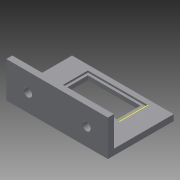
# Autodesk Inventor part: sampleholderdraft5
Saved by Autodesk Inventor 2014 SP1 (Build 180222100, 222)
## iProperties
Created: 2014-06-06
Part Number: sampleholderdraft5
Material: Generic
Document SubType Name: Modeling
Designer: miles90
Density: 1 g/cm^3
Appearance: Default
Author: miles90
Autodesk Inventor part; units mm, degrees
ref_plane "YZ Plane" through (0, 0, 0) normal (1, 0, 0) x (0, 1, 0)
ref_plane "XZ Plane" through (0, 0, 0) normal (0, 1, 0) x (-1, 0, 0)
ref_plane "XY Plane" through (0, 0, 0) normal (0, 0, 1) x (1, 0, 0)
sketch "Sketch1" plane through (0, 0, 0) normal (0, 1, 0) x (-1, 0, 0)
  line L0 (52.3087, -21.6726) -> (-32.6913, -21.6726)
  line L1 (-32.6913, -21.6726) -> (-32.6913, 38.3274)
  line L2 (-32.6913, 38.3274) -> (52.3087, 38.3274)
  line L3 (52.3087, 38.3274) -> (52.3087, -21.6726)
  dimension "d4" = 60
  dimension "d5" = 85
  constraints: 8 end point, 2 parallel, 1 horizontal, 1 perpendicular
  measures "d4" distance of L2.end L0.start
  measures "d5" distance of L0.start L0.end
extrude "Extrusion1" add sketch "Sketch1" along normal blind 20
sketch "Sketch2" plane through (0, 20, 0) normal (0, 1, 0) x (1, 0, 0)
  line L0 (32.6913, 21.6726) -> (-52.3087, 21.6726) projected
  line L1 (-52.3087, 21.6726) -> (-52.3087, -38.3274) projected
  line L2 (-52.3087, -38.3274) -> (32.6913, -38.3274) projected
  line L3 (32.6913, -38.3274) -> (32.6913, 21.6726) projected
  line L4 (-52.3087, 16.6726) -> (32.6913, 16.6726)
  line L5 (32.6913, 16.6726) -> (32.6913, -33.3274)
  line L6 (32.6913, -33.3274) -> (-52.3087, -33.3274)
  line L7 (-52.3087, -33.3274) -> (-52.3087, 16.6726)
  point P0 (0, 0)
  dimension "d8" = 0
  dimension "d9" = 0
  dimension "d10" = 5
  dimension "d11" = 5
  constraints: 8 end point, 2 parallel, 1 horizontal, 1 perpendicular
  measures "d8" distance between parallel lines of L1 L7
  measures "d9" distance between parallel lines of L5 L3
  measures "d10" distance between parallel lines of L6 L2
  measures "d11" distance between parallel lines of L0 L4
extrude "Extrusion2" cut sketch "Sketch2" against normal blind 15 contours L3 L6 L1 L4
sketch "Sketch3" plane through (0, 5, 0) normal (0, 1, 0) x (1, 0, 0)
  line L0 (-52.3087, 16.6726) -> (32.6913, 16.6726) projected
  line L1 (-52.3087, -33.3274) -> (-52.3087, 16.6726) projected
  line L2 (32.6913, -33.3274) -> (-52.3087, -33.3274) projected
  line L3 (32.6913, 16.6726) -> (32.6913, -33.3274) projected
  line L4 (-34.8087, 12.4226) -> (15.1913, 12.4226)
  line L5 (15.1913, 12.4226) -> (15.1913, -11.3274)
  line L6 (15.1913, -11.3274) -> (-34.8087, -11.3274)
  line L7 (-34.8087, -11.3274) -> (-34.8087, 12.4226)
  point P0 (0, 0)
  dimension "d14" = 17.5
  dimension "d15" = 17.5
  dimension "d16" = 4.25
  dimension "d17" = 22
  constraints: 8 end point, 2 parallel, 1 horizontal, 1 perpendicular
  measures "d14" distance between parallel lines of L3 L5
  measures "d15" distance between parallel lines of L1 L7
  measures "d16" distance between parallel lines of L4 L0
  measures "d17" distance between parallel lines of L6 L2
extrude "Extrusion3" cut sketch "Sketch3" against normal blind 1.5 contours L4 L5 L6 L7
sketch "Sketch4" plane through (0, 3.5, 0) normal (0, 1, 0) x (1, 0, 0)
  line L0 (-34.8087, 12.4226) -> (15.1913, 12.4226) projected
  line L1 (-34.8087, -11.3274) -> (-34.8087, 12.4226) projected
  line L2 (15.1913, -11.3274) -> (-34.8087, -11.3274) projected
  line L3 (15.1913, 12.4226) -> (15.1913, -11.3274) projected
  line L4 (-32.8087, 10.4226) -> (11.1913, 10.4226)
  line L5 (11.1913, 10.4226) -> (11.1913, -9.3274)
  line L6 (11.1913, -9.3274) -> (-32.8087, -9.3274)
  line L7 (-32.8087, -9.3274) -> (-32.8087, 10.4226)
  point P0 (0, 0)
  dimension "d20" = 2
  dimension "d21" = 2
  dimension "d22" = 2
  dimension "d23" = 4
  constraints: 8 end point, 2 parallel, 1 horizontal, 1 perpendicular
  measures "d20" distance between parallel lines of L1 L7
  measures "d21" distance between parallel lines of L0 L4
  measures "d22" distance between parallel lines of L2 L6
  measures "d23" distance between parallel lines of L3 L5
extrude "Extrusion4" cut sketch "Sketch4" against normal blind 1 contours L4 L5 L6 L7
sketch "Sketch5" plane through (0, 20, 0) normal (0, 1, 0) x (1, 0, 0)
  line L0 (32.6913, -33.3274) -> (-52.3087, -33.3274) projected
  line L1 (-52.3087, -33.3274) -> (-52.3087, -38.3274) projected
  line L2 (-52.3087, -38.3274) -> (32.6913, -38.3274) projected
  line L3 (32.6913, -38.3274) -> (32.6913, -33.3274) projected
  line L4 (-52.3087, -33.3274) -> (32.6913, -33.3274)
  line L5 (32.6913, -33.3274) -> (32.6913, -38.3274)
  line L6 (32.6913, -38.3274) -> (-52.3087, -38.3274)
  line L7 (-52.3087, -38.3274) -> (-52.3087, -33.3274)
  point P0 (0, 0)
  dimension "d26" = 0
  dimension "d27" = 0
  dimension "d28" = 0
  dimension "d29" = 0
  constraints: 8 end point, 2 parallel, 1 horizontal, 1 perpendicular
  measures "d26" distance between parallel lines of L0 L4
  measures "d27" distance between parallel lines of L2 L6
  measures "d28" distance between parallel lines of L3 L5
  measures "d29" distance between parallel lines of L1 L7
extrude "Extrusion5" add sketch "Sketch5" against normal blind 35
sketch "Sketch6" plane through (0, 20, 0) normal (0, 1, 0) x (1, 0, 0)
  line L0 (-52.3087, 16.6726) -> (32.6913, 16.6726) projected
  line L1 (32.6913, 16.6726) -> (32.6913, 21.6726) projected
  line L2 (32.6913, 21.6726) -> (-52.3087, 21.6726) projected
  line L3 (-52.3087, 21.6726) -> (-52.3087, 16.6726) projected
  line L4 (-52.3087, 21.6726) -> (32.6913, 21.6726)
  line L5 (32.6913, 21.6726) -> (32.6913, 16.6726)
  line L6 (32.6913, 16.6726) -> (-52.3087, 16.6726)
  line L7 (-52.3087, 16.6726) -> (-52.3087, 21.6726)
  point P0 (0, 0)
  dimension "d32" = 0
  dimension "d33" = 0
  dimension "d34" = 0
  dimension "d35" = 0
  constraints: 8 end point, 2 parallel, 1 horizontal, 1 perpendicular
  measures "d32" distance between parallel lines of L2 L4
  measures "d33" distance between parallel lines of L0 L6
  measures "d34" distance between parallel lines of L3 L7
  measures "d35" distance between parallel lines of L1 L5
extrude "Extrusion6" cut sketch "Sketch6" against normal blind 20
sketch "Sketch8" plane through (0, 20, 0) normal (0, 1, 0) x (1, 0, 0)
  line L0 (32.6913, -33.3274) -> (-52.3087, -33.3274) projected
  line L1 (-52.3087, -33.3274) -> (-52.3087, -38.3274) projected
  line L2 (-52.3087, -38.3274) -> (32.6913, -38.3274) projected
  line L3 (32.6913, -38.3274) -> (32.6913, -33.3274) projected
  line L4 (-52.3087, -33.3274) -> (32.6913, -33.3274)
  line L5 (32.6913, -33.3274) -> (32.6913, -38.3274)
  line L6 (32.6913, -38.3274) -> (-52.3087, -38.3274)
  line L7 (-52.3087, -38.3274) -> (-52.3087, -33.3274)
  point P0 (0, 0)
  dimension "d41" = 0
  dimension "d42" = 0
  dimension "d43" = 0
  dimension "d44" = 0
  constraints: 8 end point, 2 parallel, 1 horizontal, 1 perpendicular
  measures "d41" distance between parallel lines of L3 L5
  measures "d42" distance between parallel lines of L1 L7
  measures "d43" distance between parallel lines of L2 L6
  measures "d44" distance between parallel lines of L0 L4
extrude "Extrusion7" add sketch "Sketch8" along normal blind 10
sketch "Sketch9" plane through (0, -15, 0) normal (0, -1, 0) x (1, 0, 0)
  line L0 (-52.3087, 33.3274) -> (32.6913, 33.3274) projected
  line L1 (32.6913, 33.3274) -> (32.6913, 38.3274) projected
  line L2 (32.6913, 38.3274) -> (-52.3087, 38.3274) projected
  line L3 (-52.3087, 38.3274) -> (-52.3087, 33.3274) projected
  line L4 (-52.3087, 38.3274) -> (32.6913, 38.3274)
  line L5 (32.6913, 38.3274) -> (32.6913, 33.3274)
  line L6 (32.6913, 33.3274) -> (-52.3087, 33.3274)
  line L7 (-52.3087, 33.3274) -> (-52.3087, 38.3274)
  point P0 (0, 0)
  dimension "d47" = 0
  dimension "d48" = 0
  dimension "d49" = 0
  dimension "d50" = 0
  constraints: 8 end point, 2 parallel, 1 horizontal, 1 perpendicular
  measures "d47" distance between parallel lines of L2 L4
  measures "d48" distance between parallel lines of L3 L7
  measures "d49" distance between parallel lines of L0 L6
  measures "d50" distance between parallel lines of L1 L5
extrude "Extrusion8" add sketch "Sketch9" along normal blind 10
sketch "Sketch10" plane through (32.6913, 5, 33.3274) normal (0, 0, -1) x (-1, 0, 0)
  line L0 (85, 25) -> (85, 0) projected
  line L1 (0, 25) -> (85, 25) projected
  circle A0 centre (18, 9.75) radius 3.5
  circle A1 centre (67, 9.75) radius 3.5
  point P0 (32.6913, -5)
  dimension "d53" = 15.25
  dimension "d55" = 15.25
  dimension "d58" = 7
  dimension "d59" = 7
  dimension "d70" = 49
  dimension "d71" = 18
  constraints: 2 centre point
  measures "d53" distance from line of L1 A1.centre
  measures "d55" distance from line of L1 A0.centre
  measures "d58" diameter of A0
  measures "d59" diameter of A1
  measures "d70" distance of A1.centre A0.centre
  measures "d71" distance from line of L0 A1.centre
extrude "Extrusion9" cut sketch "Sketch10" against normal blind 5
sketch "Sketch11" plane through (32.6913, 0, 33.3274) normal (0, 0, -1) x (-1, 0, 0)
  line L0 (0, 0) -> (0, -25) projected
  line L1 (85, -25) -> (0, -25) projected
  line L2 (85, 0) -> (85, -25) projected
  circle A0 centre (18, -9.75) radius 3.5
  circle A1 centre (67, -9.75) radius 3.5
  point P0 (32.6913, 0)
  dimension "d62" = 18
  dimension "d63" = 18
  dimension "d64" = 7
  dimension "d65" = 7
  dimension "d66" = 15.25
  dimension "d67" = 15.25
  constraints: 2 centre point
  measures "d62" distance from line of L2 A1.centre
  measures "d63" distance from line of L0 A0.centre
  measures "d64" diameter of A0
  measures "d65" diameter of A1
  measures "d66" distance from line of L1 A0.centre
  measures "d67" distance from line of L1 A1.centre
extrude "Extrusion10" cut sketch "Sketch11" against normal blind 5
sketch "Sketch13" plane through (0, 5, 0) normal (0, 1, 0) x (1, 0, 0)
  line L0 (-52.3087, 16.6726) -> (32.6913, 16.6726) projected
  line L1 (32.6913, -33.3274) -> (-52.3087, -33.3274) projected
  line L2 (32.6913, 16.6726) -> (32.6913, -33.3274) projected
  line L3 (32.6913, 16.6726) -> (29.6913, 16.6726)
  line L4 (29.6913, 16.6726) -> (29.6913, -33.3274)
  line L5 (29.6913, -33.3274) -> (32.6913, -33.3274)
  line L6 (32.6913, -33.3274) -> (32.6913, 16.6726)
  point P0 (0, 0)
  dimension "d72" = 0
  dimension "d73" = 0
  dimension "d74" = 0
  dimension "d75" = 3
  constraints: 8 end point, 2 parallel, 1 horizontal, 1 perpendicular
  measures "d72" distance between parallel lines of L2 L6
  measures "d73" distance between parallel lines of L1 L5
  measures "d74" distance between parallel lines of L0 L3
  measures "d75" distance between parallel lines of L2 L4
extrude "Extrusion11" add sketch "Sketch13" along normal blind 20
sketch "Sketch14" plane through (32.6913, 0, 33.3274) normal (1, 0, 0) x (0, 0, -1)
  line L0 (50, 0) -> (50, 25) projected
  line L1 (50, 0) -> (0, 0) projected
  circle A0 centre (41.5, 10) radius 2
  circle A1 centre (27.5, 10) radius 2
  point P0 (33.3274, 0)
  dimension "d78" = 4
  dimension "d79" = 4
  dimension "d80" = 8.5
  dimension "d81" = 10
  dimension "d82" = 22.5
  dimension "d83" = 10
  constraints: 2 centre point
  measures "d78" diameter of A1
  measures "d79" diameter of A0
  measures "d80" distance from line of L0 A0.centre
  measures "d81" distance from line of L1 A0.centre
  measures "d82" distance from line of L0 A1.centre
  measures "d83" distance from line of L1 A1.centre
extrude "Extrusion12" cut sketch "Sketch14" against normal blind 5
sketch "Sketch15" plane through (0, -25, 0) normal (0, -1, 0) x (1, 0, 0)
  line L0 (-52.3087, 33.3274) -> (32.6913, 33.3274) projected
  line L1 (32.6913, 33.3274) -> (32.6913, 38.3274) projected
  line L2 (32.6913, 38.3274) -> (-52.3087, 38.3274) projected
  line L3 (-52.3087, 38.3274) -> (-52.3087, 33.3274) projected
  line L4 (-52.3087, 38.3274) -> (32.6913, 38.3274)
  line L5 (32.6913, 38.3274) -> (32.6913, 33.3274)
  line L6 (32.6913, 33.3274) -> (-52.3087, 33.3274)
  line L7 (-52.3087, 33.3274) -> (-52.3087, 38.3274)
  point P0 (0, 0)
  dimension "d86" = 0
  dimension "d87" = 0
  dimension "d88" = 0
  dimension "d89" = 0
  constraints: 8 end point, 2 parallel, 1 horizontal, 1 perpendicular
  measures "d86" distance between parallel lines of L2 L4
  measures "d87" distance between parallel lines of L0 L6
  measures "d88" distance between parallel lines of L3 L7
  measures "d89" distance between parallel lines of L1 L5
extrude "Extrusion13" cut sketch "Sketch15" against normal blind 25
sketch "Sketch16" plane through (15.1913, 5, -12.4226) normal (-1, 0, 0) x (0, 0, 1)
  line L0 (0, 0) -> (23.75, 0) projected
  line L1 (0, 0) -> (0, -1.5) projected
  line L2 (0, -1.5) -> (23.75, -1.5) projected
  line L3 (23.75, 0) -> (23.75, -1.5) projected
  point P0 (12.4226, -5)
sketch "Sketch17" plane through (0, 2.5, 0) normal (0, 1, 0) x (1, 0, 0)
  line L0 (-32.8087, 10.4226) -> (11.1913, 10.4226) projected
  line L1 (-32.8087, -9.3274) -> (-32.8087, 10.4226) projected
  line L2 (11.1913, -9.3274) -> (-32.8087, -9.3274) projected
  line L3 (11.1913, 10.4226) -> (11.1913, -9.3274) projected
  line L4 (-32.8087, 10.4226) -> (11.1913, 10.4226)
  line L5 (11.1913, 10.4226) -> (11.1913, -9.3274)
  line L6 (11.1913, -9.3274) -> (-32.8087, -9.3274)
  line L7 (-32.8087, -9.3274) -> (-32.8087, 10.4226)
  point P0 (0, 0)
  dimension "d93" = 0
  dimension "d94" = 0
  dimension "d95" = 0
  dimension "d96" = 0
  constraints: 8 end point, 2 parallel, 1 horizontal, 1 perpendicular
  measures "d93" distance between parallel lines of L0 L4
  measures "d94" distance between parallel lines of L3 L5
  measures "d95" distance between parallel lines of L1 L7
  measures "d96" distance between parallel lines of L2 L6
extrude "Extrusion14" cut sketch "Sketch17" along normal mid plane 5
sketch "Sketch18" plane through (0, 25, 0) normal (0, 1, 0) x (1, 0, 0)
  line L0 (32.6913, 16.6726) -> (29.6913, 16.6726) projected
  line L1 (29.6913, 16.6726) -> (29.6913, -33.3274) projected
  line L2 (32.6913, -33.3274) -> (29.6913, -33.3274) projected
  line L3 (32.6913, -33.3274) -> (32.6913, 16.6726) projected
  line L4 (29.6913, 16.6726) -> (32.6913, 16.6726)
  line L5 (32.6913, 16.6726) -> (32.6913, -33.3274)
  line L6 (32.6913, -33.3274) -> (29.6913, -33.3274)
  line L7 (29.6913, -33.3274) -> (29.6913, 16.6726)
  point P0 (0, 0)
  dimension "d99" = 0
  dimension "d100" = 0
  dimension "d101" = 0
  dimension "d102" = 0
  constraints: 8 end point, 2 parallel, 1 horizontal, 1 perpendicular
  measures "d99" distance between parallel lines of L3 L5
  measures "d100" distance between parallel lines of L1 L7
  measures "d101" distance between parallel lines of L2 L6
  measures "d102" distance between parallel lines of L0 L4
extrude "Extrusion15" cut sketch "Sketch18" against normal blind 20
body "Solid1"
